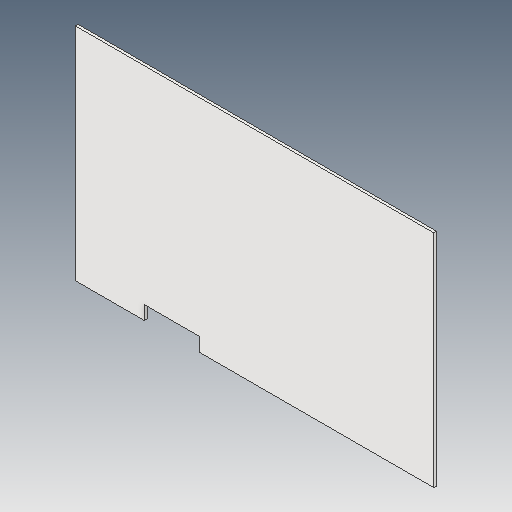
# Autodesk Inventor part: 防水p2
Saved by Autodesk Inventor 2020.3 (Build 243373000, 373)
## iProperties
Part Number: 防水p2
Material: 一般
Document SubType Name: Modeling
Designer: highs
Density: 1 g/cm^3
Appearance: 既定
Author: highs
Autodesk Inventor part; units mm, degrees
ref_plane "YZ Plane" through (0, 0, 0) normal (1, 0, 0) x (0, 1, 0)
ref_plane "XZ Plane" through (0, 0, 0) normal (0, 1, 0) x (-1, 0, 0)
ref_plane "XY Plane" through (0, 0, 0) normal (0, 0, 1) x (1, 0, 0)
sketch "スケッチ1" plane through (0, 0, 0) normal (0, 0, 1) x (1, 0, 0)
  line L0 (0, 0) -> (100, 0)
  line L1 (100, 0) -> (100, 20)
  line L2 (100, 20) -> (180, 20)
  line L3 (180, 20) -> (180, 0)
  line L4 (180, 0) -> (520, 0)
  line L5 (520, 0) -> (520, 320)
  line L6 (520, 320) -> (0, 320)
  line L7 (0, 320) -> (0, 0)
  dimension "d0" = 520
  dimension "d1" = 320
  dimension "d2" = 20
  dimension "d3" = 80
  dimension "d4" = 100
  constraints: 16 end point, 6 perpendicular, 2 point on line, 1 horizontal
  measures "d0" distance of L5.end L6.end
  measures "d1" distance of L6.end L0.start
  measures "d2" distance of L0.end L1.end
  measures "d3" distance of L1.end L2.end
  measures "d4" distance of L0.start L0.end
extrude "押し出し1" add sketch "スケッチ1" along normal blind 4
